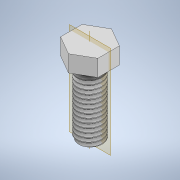
# Autodesk Inventor part: threadExample
Saved by Autodesk Inventor 2021 (Build 250183000, 183)
## iProperties
Created: 2020-06-13
Part Number: threadExample
Material: Generic
Document SubType Name: Modeling
Designer: robst
Density: 1 g/cm^3
Appearance: Default
Author: robst
Autodesk Inventor part; units mm, degrees
ref_plane "YZ Plane" through (0, 0, 0) normal (1, 0, 0) x (0, 1, 0)
ref_plane "XZ Plane" through (0, 0, 0) normal (0, 1, 0) x (-1, 0, 0)
sketch "Sketch1" plane through (0, 0, 0) normal (0, 1, 0) x (-1, 0, 0)
  circle A0 centre (0, 0) radius 4.746
  dimension "d0" = 9.492
  constraints: 1 centre point, 1 coincident
  measures "d0" diameter of A0
extrude "Extrusion1" add sketch "Sketch1" against normal blind 25.4
sketch "Sketch14" plane through (0, 0, 0) normal (0, 1, 0) x (1, 0, 0)
  line L0 (0, 8.2489) -> (7.1437, 4.1244)
  line L1 (7.1437, 4.1244) -> (7.1437, -4.1244)
  line L2 (7.1437, -4.1244) -> (0, -8.2489)
  line L3 (0, -8.2489) -> (-7.1437, -4.1244)
  line L4 (-7.1437, -4.1244) -> (-7.1438, 4.1244)
  line L5 (-7.1438, 4.1244) -> (0, 8.2489)
  point P0 (0, 0)
  point P1 (0, 0)
  dimension "d149" = 14.2875
  constraints: 12 end point, 1 coincident, 1 vertical, 13 other
  measures "d149" distance between parallel lines of L1 L4
extrude "Extrusion3" add sketch "Sketch14" along normal blind 6.35
sketch "Sketch15" plane through (0, 0, 0) normal (0, 0, 1) x (1, 0, 0)
  line L0 (4.746, 0) -> (4.746, -25.4) projected
  line L1 (-4.746, -25.4) -> (4.746, -25.4) projected
  line L2 (4.746, -25.0522) -> (4.746, -25.4) construction
  line L3 (0, -32.0291) -> (0, 5.3382) projected
  line L4 (4.746, -25.4) -> (3.7998, -25.9463)
  line L5 (3.7998, -25.9463) -> (3.7998, -26.1447)
  line L6 (3.7998, -26.1447) -> (4.746, -26.691)
  line L7 (4.746, -26.691) -> (4.746, -25.4)
  point P0 (0, 0)
  point P1 (4.746, -24.8537)
  dimension "d167" = 60
  dimension "d168" = 60
  dimension "d169" = 0.1984
  dimension "d170" = 3.7998
  dimension "d171" = 0
  dimension "d172" = 60
  constraints: 10 end point, 2 vertical, 1 parallel, 1 point on line
  measures "d167" angle of L6 L4
  measures "d168" angle of L7 L4
  measures "d169" distance of L5.end L4.end
  measures "d170" distance between parallel lines of L5 L3
  measures "d171" distance from line of L2.end L1
  measures "d172" angle of L7 L6
coil "Coil13" sketch "Sketch15" operation cut axis through (0, -10, 0) along (0, 1, 0) pitch 1.5875 turns 16 hand right
body "Solid1"
